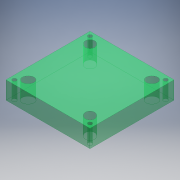
# Autodesk Inventor part: PCB_Camera
Saved by Autodesk Inventor 2016 (Build 200138000, 138)
## iProperties
Created: 2016-04-14
Part Number: PCB_Camera
Material: Generic
Document SubType Name: Modeling
Designer: Andres
Density: 1 g/cm^3
Appearance: Clear - Green 1
Author: Andres
Autodesk Inventor part; units mm, degrees
ref_plane "YZ Plane" through (0, 0, 0) normal (1, 0, 0) x (0, 1, 0)
ref_plane "XZ Plane" through (0, 0, 0) normal (0, 1, 0) x (-1, 0, 0)
ref_plane "XY Plane" through (0, 0, 0) normal (0, 0, 1) x (1, 0, 0)
sketch "Sketch1" plane through (0, 0, 0) normal (0, 0, 1) x (1, 0, 0)
  line L0 (-19, 19) -> (19, 19)
  line L1 (19, 19) -> (19, -19)
  line L2 (19, -19) -> (-19, -19)
  line L3 (-19, -19) -> (-19, 19)
  point P0 (0, 0)
  point P1 (0, 19)
  point P2 (-19, 0)
  dimension "d0" = 38
  dimension "d1" = 38
  constraints: 8 end point, 2 midpoint, 2 parallel, 1 horizontal, 1 horizontal alignment, 1 perpendicular, 1 vertical alignment
  measures "d0" distance of L0.end L1.end
  measures "d1" distance of L1.end L2.end
extrude "Extrusion1" add sketch "Sketch1" along normal blind 8
sketch "Sketch2" plane through (0, 0, 8) normal (0, 0, 1) x (1, 0, 0)
  circle A0 centre (-17.1, 17.1) radius 0.9
  circle A1 centre (17.1, 17.1) radius 0.9
  circle A2 centre (-17.1, -17.1) radius 0.9
  circle A3 centre (17.1, -17.1) radius 0.9
  line L0 (19, 19) -> (-19, 19) projected
  line L1 (-19, 19) -> (-19, -19) projected
  line L2 (19, -19) -> (19, 19) projected
  line L3 (-19, -19) -> (19, -19) projected
  ellipse E0 centre (-14, -14) end of major axis (-15.5556, -12.4444) minor radius 2.55
  ellipse E1 centre (-14, 14) end of major axis (-12.2322, 12.2322) minor radius 2.2
  ellipse E2 centre (14, 14) end of major axis (12.2322, 12.2322) minor radius 2.2
  ellipse E3 centre (14, -14) end of major axis (12.2322, -12.2322) minor radius 2.2
  point P0 (0, 0)
  dimension "d24" = 2.2
  dimension "d29" = 2.55
  dimension "d30" = 2.5
  dimension "d31" = 2.2
  dimension "d36" = 2.2
  dimension "d37" = 2.5
  dimension "d38" = 2.5
  dimension "d39" = 2.2
  dimension "d4" = 1.8
  dimension "d5" = 1.8
  dimension "d6" = 1.8
  dimension "d7" = 1.8
  dimension "d8" = 1
  dimension "d9" = 1.9
  dimension "d10" = 1.9
  dimension "d11" = 1.9
  dimension "d12" = 1.9
  dimension "d13" = 1.9
  dimension "d14" = 1.9
  dimension "d15" = 1.9
  dimension "d27" = 14
  dimension "d28" = 14
  dimension "d32" = 14
  dimension "d33" = 14
  dimension "d34" = 14
  dimension "d35" = 14
  dimension "d40" = 14
  dimension "d41" = 14
  constraints: 4 centre point, 8 other
  measures "d4" diameter of A0
  measures "d5" diameter of A1
  measures "d6" diameter of A2
  measures "d7" diameter of A3
  measures "d8" distance edge to line of A0 L0
  measures "d9" distance from line of L1 A0.centre
  measures "d10" distance from line of L2 A1.centre
  measures "d11" distance from line of L0 A1.centre
  measures "d12" distance from line of L2 A3.centre
  measures "d13" distance from line of L3 A3.centre
  measures "d14" distance from line of L3 A2.centre
  measures "d15" distance from line of L1 A2.centre
  measures "d27" horizontal distance of point (0, 0) point (-14, -14)
  measures "d28" horizontal distance of point (0, 0) point (-14, -14)
  measures "d32" horizontal distance of point (-14, 14) point (0, 0)
  measures "d33" horizontal distance of point (-14, 14) point (0, 0)
  measures "d34" horizontal distance of point (14, 14) point (0, 0)
  measures "d35" horizontal distance of point (14, 14) point (0, 0)
  measures "d40" horizontal distance of point (0, 0) point (14, -14)
  measures "d41" horizontal distance of point (0, 0) point (14, -14)
hole "Hole1" at (-17.1, 17.1, 8) at (17.1, 17.1, 8) at (17.1, -17.1, 8) at (-17.1, -17.1, 8) direction (0, 0, -1) diameter 1.8 end through all
extrude "Extrusion2" cut sketch "Sketch2" against normal blind 8 contours E0 | E1 | E2 | E3
body "Solid1"
